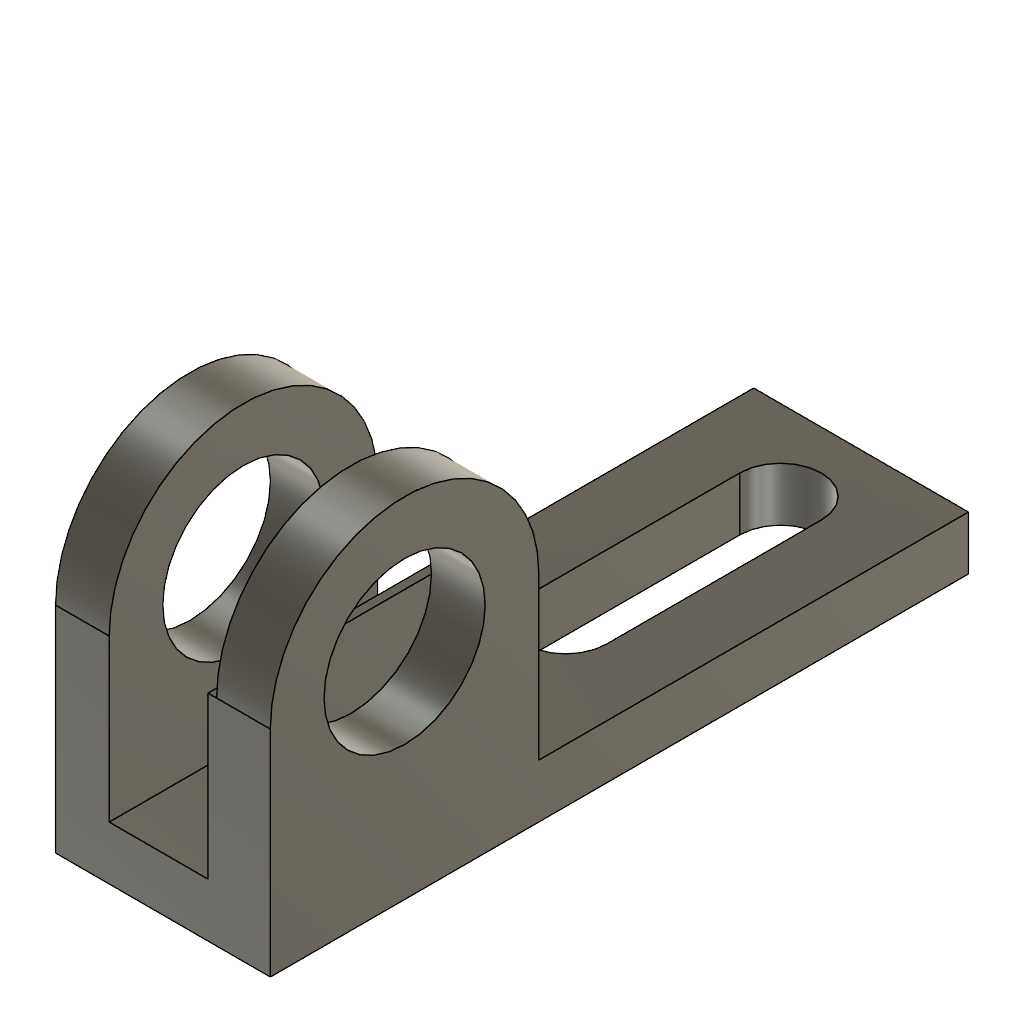
exercise 5 (Autodesk Fusion 360 design; units mm, degrees)
part number: 2026-10-01-22-51-15-792
Autodesk Fusion 360 part; units mm, degrees
note: some values were not read from the file. Set by a fixed rule: which sketch regions a step uses.
sketch "Sketch1" plane through (0, 0, 0) normal (0, 1, 0) x (1, 0, 0)
  line L0 (0, 0) -> (-40, 0)
  line L1 (-40, 0) -> (-40, -40)
  line L2 (0, -40) -> (0, 0)
  line L3 (-40, -40) -> (-30, -40)
  line L4 (-30, -40) -> (-30, -10)
  line L5 (-30, -10) -> (-11.6065, -10)
  line L6 (-11.6065, -10) -> (-11.6065, -40)
  line L7 (-11.6065, -40) -> (0, -40)
  dimension "d6" = 40
  dimension "d7" = 40
  dimension "d8" = 10
  dimension "d9" = 11.6065
  dimension "d10" = 10
  constraint horizontal L0
  constraint vertical L1
  constraint vertical L2
  constraint coincident L0.start L2.end
  constraint perpendicular L1 L3
  constraint perpendicular L3 L4
  constraint perpendicular L1 L5
  constraint perpendicular L5 L6
  constraint perpendicular L2 L7
  measures "d6" distance of L0.start L0.end
  measures "d7" distance of L0.end L1.end
  measures "d8" distance of L1.end L3.end
  measures "d9" distance of L2.start L6.end
  measures "d10" distance of L0 L5
extrude "Extrude1" add sketch "Sketch1" along normal blind 130
sketch "Sketch2" plane through (-40, 0, 0) normal (-1, 0, 0) x (0, -1, 0)
  line L0 (0, 0) -> (0, 40)
  line L1 (0, 40) -> (-130, 40)
  line L2 (-130, 40) -> (-130, 0)
  line L3 (-130, 0) -> (0, 0)
  circle A0 centre (-25, 40) radius 15
  arc A1 (0, 40) -> (-50, 40) centre (-25, 40) ccw
  line L4 (-50, 40) -> (-50, 10)
  line L5 (-50, 10) -> (-130, 10)
  dimension "d13" = 50
  dimension "d14" = 30
  dimension "d15" = 25
  dimension "d16" = 30
  constraint coincident L1 A0.centre
  constraint concentric A0 A1
  constraint coincident L1 A1.end
  constraint tangent A1 L4
  constraint coincident L2 L5.end
  constraint perpendicular L2 L5
  measures "d13" diameter of A1
  measures "d14" diameter of A0
  measures "d15" distance of L0.end A0.centre
  measures "d16" distance of A1.end L4.end
extrude "Extrude2" add sketch "Sketch2" against normal blind 10 contours L1 A0 A1
extrude "Extrude3" cut sketch "Sketch2" against normal blind 10 contours L1 A0 | L1 A0
extrude "Extrude4" cut sketch "Sketch2" against normal blind 10 contours L1 L2 L4 L5
extrude "Extrude5" add sketch "Sketch2" against normal blind 10 contours L1 L2 L4 L5
sketch "Sketch3" plane through (-40, 0, 0) normal (-1, 0, 0) x (0, -1, 0)
  line L0 (-130, 10) -> (-130, 0)
  line L1 (-130, 0) -> (0, 0)
  line L2 (0, 0) -> (0, 40)
  constraint vertical L0
  constraint coincident L1.end L2.start
  constraint perpendicular L0 L1
  constraint perpendicular L1 L2
extrude "Extrude6" cut sketch "Sketch2" against normal blind 66.91 contours L1 L2 L4 L5
sketch "Sketch4" plane through (0, 0, 0) normal (1, 0, 0) x (0, 1, 0)
  line L0 (130, 10) -> (50, 10)
  line L1 (50, 10) -> (50, 40)
  line L2 (50, 40) -> (0, 40)
  line L3 (0, 40) -> (0, 0)
  line L4 (0, 0) -> (130, 0)
  line L5 (130, 0) -> (130, 10)
  circle A0 centre (25, 40) radius 15
  arc A1 (50, 40) -> (0, 40) centre (25, 40) ccw
  dimension "d27" = 50
  dimension "d28" = 30
  constraint midpoint L2 A0.centre
  constraint concentric A0 A1
  measures "d27" diameter of A1
  measures "d28" diameter of A0
extrude "Extrude7" cut sketch "Sketch4" against normal blind 10 contours L2 A0 A1 | L2 A0 | L2 A0
extrude "Extrude8" add sketch "Sketch4" against normal blind 10 contours L2 A0 A1
sketch "Sketch5" plane through (0, 0, 10) normal (0, 0, 1) x (-1, 0, 0)
  line L0 (30, -50) -> (30, 0)
  line L1 (30, 0) -> (11.6065, 0)
  line L2 (11.6065, 0) -> (11.6065, -50)
  line L3 (11.6065, -50) -> (0, -50)
  line L4 (0, -50) -> (0, -130)
  line L5 (0, -130) -> (40, -130)
  line L6 (40, -130) -> (40, -50)
  line L7 (40, -50) -> (30, -50)
  line L8 (12.4119, -75) -> (12.4119, -115)
  arc A0 (12.4119, -115) -> (27.5881, -115) centre (20, -115) ccw
  line L9 (27.5881, -115) -> (27.5881, -75)
  arc A1 (27.5881, -75) -> (12.4119, -75) centre (20, -75) ccw
  line L10 (20, -75) -> (20, -115) construction
  point P0 (20, -95)
  dimension "d33" = 40
  constraint tangent L8 A0
  constraint tangent A0 L9
  constraint parallel L8 L9
  constraint tangent L9 A1
  constraint tangent L8 A1
  constraint vertical L10
  constraint midpoint L10 P0
  measures "d33" distance of A1.centre A0.centre
extrude "Extrude9" cut sketch "Sketch5" against normal blind 34.041 contours L8 A0 L9 A1
